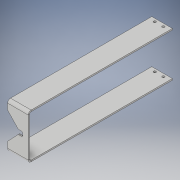
# Autodesk Inventor part: guidebar
Saved by Autodesk Inventor 2017 (Build 210142000, 142)
## iProperties
Created: 2017-02-05
Part Number: guidebar
Material: Generic
Document SubType Name: Sheet Metal
Designer: kingb
Density: 1 g/cm^3
Sheet Metal Rule: Default
Appearance: Default
Flat Pattern Width: 4.34864 cm
Flat Pattern Length: 69.3747 cm
Flat Pattern Area: 301.685 cm^2
Sheet Metal Width: 1.712 in
Sheet Metal Length: 27.313 in
Sheet Metal Area: 46.761 in^2
Author: kingb
Autodesk Inventor part; units mm, degrees
ref_plane "YZ Plane" through (0, 0, 0) normal (1, 0, 0) x (0, 1, 0)
ref_plane "XZ Plane" through (0, 0, 0) normal (0, 1, 0) x (-1, 0, 0)
ref_plane "XY Plane" through (0, 0, 0) normal (0, 0, 1) x (1, 0, 0)
sketch "Sketch1" plane through (0, 0, 0) normal (0, 0, 1) x (1, 0, 0)
  line L0 (0, 3.048) -> (-43.4864, 3.048) construction
  line L1 (-43.4864, 0) -> (-43.4864, 3.048)
  line L2 (-43.4864, 0) -> (0, 0)
  line L3 (0, 0) -> (0, 3.048)
  line L4 (0, 88.646) -> (-43.4864, 88.646)
  line L5 (-43.4864, 85.598) -> (-43.4864, 88.646)
  line L6 (-43.4864, 85.598) -> (0, 85.598) construction
  line L7 (0, 85.598) -> (0, 88.646)
  line L8 (0, 0) -> (-43.4864, 0)
  line L9 (-43.4864, 0) -> (-43.4864, 88.646)
  line L10 (-43.4864, 88.646) -> (0, 88.646)
  line L11 (0, 88.646) -> (0, 0)
extrude "Plate1" add sketch "Sketch1" along normal blind 3.048
sketch "Sketch2" plane through (-43.4864, 0, 0) normal (0, -1, 0) x (1, 0, 0)
  line L0 (43.4864, 0) -> (0, 0)
  line L1 (0, 0) -> (0, -301.752)
  line L2 (0, -301.752) -> (43.4864, -301.752)
  line L3 (43.4864, -301.752) -> (43.4864, 0)
  constraints: 6 end point, 1 horizontal, 1 perpendicular, 1 vertical
edge flange "Flange1" height 304.8 angle 90 thickness 3.048 bend radius 3.048 thickness toward (0, -1, 0) relief straight relief width 3.048 relief depth 1.524 corner gap 3.048 corner form 0 edges at (-21.7432, 0, 0) (-21.7432, 88.646, 0) wall of the first edge with corners at (0, 0, 0) (-43.4864, 0, 0) (-43.4864, 0, -301.752) (0, 0, -301.752)
bend "Bend1"
corner "Corner1"
sketch "Sketch3" plane through (0, 0, 3.048) normal (0, 0, 1) x (1, 0, 0)
  line L0 (-43.4864, 3.048) -> (-43.4864, 15.748) construction
  line L1 (-43.4864, 15.748) -> (-21.8429, 38.5703)
  line L2 (-16.3873, 44.323) -> (-20.9038, 49.0855) construction
  line L3 (-43.4864, 85.598) -> (-43.4864, 72.898) construction
  line L4 (-43.4864, 3.048) -> (-43.4864, 85.598) projected
  line L5 (-43.4864, 72.898) -> (-43.4864, 15.748)
  line L6 (-19.5391, 49.0855) -> (-14.5538, 49.0855)
  line L7 (-11.3788, 45.9105) -> (-11.3788, 42.7355)
  line L8 (-14.5538, 39.5605) -> (-19.5391, 39.5605)
  line L9 (-20.9038, 39.5605) -> (-16.3873, 44.323) construction
  line L10 (-21.8429, 50.0757) -> (-43.4864, 72.898)
  arc A0 (-14.5538, 39.5605) -> (-11.3788, 42.7355) centre (-14.5538, 42.7355) ccw
  arc A1 (-11.3788, 45.9105) -> (-14.5538, 49.0855) centre (-14.5538, 45.9105) ccw
  arc A2 (-21.8429, 50.0757) -> (-19.5391, 49.0855) centre (-19.5391, 52.2605) ccw
  arc A3 (-19.5391, 39.5605) -> (-21.8429, 38.5703) centre (-19.5391, 36.3855) ccw
  line L11 (-43.4864, 3.048) -> (-43.4864, 85.598) projected
  point P0 (0, 0)
  point P1 (-11.3788, 49.0855)
  point P2 (-11.3788, 39.5605)
  dimension "d11" = 12.7
  dimension "d12" = 28.575
  dimension "d14" = 12.7
  dimension "d18" = 9.525
  dimension "d19" = 9.525
  dimension "d20" = 9.525
  dimension "d24" = 3.175
  dimension "d25" = 11.5054
  constraints: 20 end point, 8 point on circle, 8 point on line, 8 tangent, 4 centre point, 4 collinear, 3 equal radius, 2 perpendicular, 1 horizontal
  measures "d11" distance of L0.start L0.end
  measures "d12" vertical distance of L3.end L2.start
  measures "d14" distance of L3.end L3.start
  measures "d18" distance of L2.end point (-11.379, 49.085)
  measures "d19" distance of point (-11.379, 49.085) point (-11.379, 39.56)
  measures "d20" distance of point (-11.379, 39.56) L9.start
  measures "d24" radius of A0
  measures "d25" distance of L1.end L10.start
extrude "Extrusion1" cut sketch "Sketch3" against normal up to next
sketch "Sketch4" plane through (-43.4864, -3.048, -301.752) normal (0, -1, 0) x (1, 0, 0)
  circle A0 centre (12.7, 6.35) radius 2.54
  circle A1 centre (30.7864, 6.35) radius 2.54
  line L0 (0, 0) -> (0, 298.704) projected
  line L1 (43.4864, 0) -> (0, 0) projected
  line L2 (43.4864, 0) -> (43.4864, 298.704) projected
  point P0 (43.4864, 301.752)
  dimension "d26" = 5.08
  dimension "d27" = 5.08
  dimension "d28" = 12.7
  dimension "d29" = 6.35
  dimension "d30" = 6.35
  dimension "d31" = 12.7
  constraints: 2 centre point
  measures "d26" diameter of A0
  measures "d27" diameter of A1
  measures "d28" distance from line of L0 A0.centre
  measures "d29" distance from line of L1 A0.centre
  measures "d30" distance from line of L1 A1.centre
  measures "d31" distance from line of L2 A1.centre
extrude "Extrusion2" cut sketch "Sketch4" against normal up to surface (94.742 mm away)
equation "\"d1\" = BendReliefWidth"
equation "\"d2\" = BendReliefDepth"
equation "\"d3\" = MinimumRemnant"
equation "\"d4\" = BendRadius"
equation "\"d7\" = BendRadius"
equation "\"d8\" = CornerReliefSize"
equation "\"d9\" = GapSize"
equation "\"d10\" = JacobiRadiusSize"
equation "\"BendRadius\" = Thickness"
equation "\"BendReliefWidth\" = Thickness"
equation "\"BendReliefDepth\" = 0.5 * Thickness"
equation "\"CornerReliefSize\" = 4 * Thickness"
equation "\"MinimumRemnant\" = 2 * Thickness"
equation "\"TransitionRadius\" = BendRadius"
equation "\"JacobiRadiusSize\" = BendRadius"
equation "\"GapSize\" = Thickness"
equation "\"d0\" = BendRadius"
equation "\"Thickness\" = 3.048"
body "Solid1"
